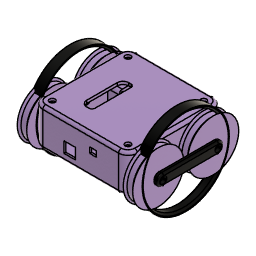
Bug (Autodesk Fusion 360 design; units mm, degrees)
Autodesk Fusion 360 part; units mm, degrees
sketch "Sketch1" plane through (0, 0, 0) normal (0, 0, 1) x (1, 0, 0)
  line L0 (-40, 50) -> (40, 50)
  line L1 (50, 40) -> (50, -40)
  line L2 (40, -50) -> (-40, -50)
  line L3 (-50, -40) -> (-50, 40)
  line L4 (-50, 0) -> (0, 0) construction
  line L5 (0, 50) -> (0, 0) construction
  arc A0 (-40, 50) -> (-50, 40) centre (-40, 40) ccw
  arc A1 (50, 40) -> (40, 50) centre (40, 40) ccw
  arc A2 (-50, -40) -> (-40, -50) centre (-40, -40) ccw
  arc A3 (40, -50) -> (50, -40) centre (40, -40) ccw
  arc A4 (47, 40) -> (40, 47) centre (40, 40) ccw
  line L6 (-40, 47) -> (40, 47)
  arc A5 (-40, 47) -> (-47, 40) centre (-40, 40) ccw
  line L7 (-47, -40) -> (-47, 40)
  arc A6 (-47, -40) -> (-40, -47) centre (-40, -40) ccw
  line L8 (40, -47) -> (-40, -47)
  arc A7 (40, -47) -> (47, -40) centre (40, -40) ccw
  line L9 (47, 40) -> (47, -40)
  circle A8 centre (23.9, -29.85) radius 1.4
  circle A9 centre (19.2, 22) radius 1.4
  circle A10 centre (-8.7, 22) radius 1.4
  circle A11 centre (-8.7, 22) radius 4
  circle A12 centre (19.2, 22) radius 4
  circle A13 centre (23.9, -29.85) radius 4
  line L10 (27.5, 47) -> (47, 27.5)
  line L11 (27.5, 47) -> (52.1887, 47) construction
  line L12 (-47, -27.5) -> (-27.5, -47)
  line L13 (-47, -27.5) -> (-27.798, -27.5) construction
  line L14 (27.5, -47) -> (47, -27.5)
  line L15 (27.5, -47) -> (53.0622, -47) construction
  line L16 (-27.5, 47) -> (-47, 27.5)
  line L17 (-27.5, 47) -> (-10.4675, 47) construction
  point P0 (-50, 50)
  point P1 (50, 50)
  point P2 (-50, -50)
  dimension "d1" = 100
  dimension "d2" = 100
  dimension "d3" = 10
  dimension "d4" = 10
  dimension "d5" = 10
  dimension "d6" = 10
  dimension "d7" = 3
  dimension "d8" = 2.8
  dimension "d9" = 2.8
  dimension "d10" = 2.8
  dimension "d11" = 20.15
  dimension "d12" = 72
  dimension "d13" = 26.1
  dimension "d14" = 30.8
  dimension "d15" = 27.9
  dimension "d16" = 8
  dimension "d17" = 8
  dimension "d18" = 8
  dimension "d19" = 45
  dimension "d20" = 45
  dimension "d21" = 45
  dimension "d22" = 135
  dimension "d23" = 22.5
  dimension "d24" = 22.5
  dimension "d25" = 22.5
  dimension "d26" = 22.5
  constraint horizontal L0
  constraint vertical L1
  constraint horizontal L2
  constraint vertical L3
  constraint coincident L4.end L5.end
  constraint vertical L5
  constraint horizontal L4
  constraint coincident L0 L5.start
  constraint coincident L3 L4.start
  constraint coincident P0 L0
  constraint coincident P0 L3
  constraint tangent L0 A0
  constraint tangent L3 A0
  constraint coincident P1 L0
  constraint coincident P1 L1
  constraint tangent L0 A1
  constraint tangent L1 A1
  constraint coincident P2 L2
  constraint coincident P2 L3
  constraint tangent L2 A2
  constraint tangent L3 A2
  constraint tangent L1 A3
  constraint tangent L2 A3
  constraint midpoint L0 L5.start
  constraint midpoint L3 L4.start
  constraint horizontal A9.centre A10.centre
  constraint concentric A10 A11
  constraint concentric A9 A12
  constraint concentric A8 A13
  constraint horizontal L11
  constraint coincident L6 L10.start
  constraint coincident L9 L10.end
  constraint horizontal L13
  constraint coincident L7 L12.start
  constraint coincident L8 L12.end
  constraint horizontal L15
  constraint coincident L8 L14.start
  constraint coincident L9 L14.end
  constraint horizontal L17
  constraint coincident L6 L16.start
  constraint coincident L7 L16.end
  measures "d1" distance of P0 P1
  measures "d2" distance of P0 P2
  measures "d3" radius of A0
  measures "d4" radius of A1
  measures "d5" radius of A2
  measures "d6" radius of A3
  measures "d8" diameter of A8
  measures "d9" diameter of A9
  measures "d10" diameter of A10
  measures "d11" distance of L2 A8.centre
  measures "d12" distance of L2 A9.centre
  measures "d13" distance of L1 A8.centre
  measures "d14" distance of L1 A9.centre
  measures "d15" distance of A9.centre A10.centre
  measures "d16" diameter of A11
  measures "d17" diameter of A12
  measures "d18" diameter of A13
  measures "d19" angle of L10 L11
  measures "d20" angle of L12 L13
  measures "d21" angle of L14 L15
  measures "d22" angle of L16 L17
  measures "d23" distance of L3 L16.start
  measures "d24" distance of L1 L10.start
  measures "d25" distance of L1 L14.start
  measures "d26" distance of L3 L12.end
extrude "Extrude2" add sketch "Sketch1" along normal blind 40 contours L0 L1 L2 L3 A0 A1 A2 A3 makes body 1
extrude "Extrude3" add sketch "Sketch1" along normal blind 3 contours L6 L7 L8 L9 L10 L12 L14 L16 bodies 1
extrude "Extrude4" add sketch "Sketch1" along normal blind 37 contours A4 L6 L9 L10 | L8 A7 L9 L14 | L6 A5 L7 L16 | L7 A6 L8 L12 bodies 1
extrude "Extrude5" add sketch "Sketch1" along normal blind 6 contours A11 | A12 | A13 bodies 1
extrude "Extrude6" add sketch "Sketch1" along normal blind 0.4 contours A8 | A9 | A10 bodies 1
fillet "Fillet3" radius 1 9 edges at (20.1707, -31.2965, 6) (22.5947, -29.3437, 6) (17.8947, 22.5063, 6) (15.4707, 20.5535, 6) (-10.0053, 22.5063, 6) (-12.4293, 20.5535, 6) (-12.4293, 23.4465, 3) (15.4707, 23.4465, 3) (20.1707, -28.4035, 3) on bodies 1
sketch "Sketch2" plane through (0, -50, 0) normal (0, -1, 0) x (1, 0, 0)
  line L0 (-40, 0) -> (40, 0)
  line L1 (40, 0) -> (40, 40)
  line L2 (40, 40) -> (-40, 40)
  line L3 (-40, 40) -> (-40, 0)
  line L4 (-17.7, 19.5) -> (-5.5, 19.5)
  line L5 (-5.5, 19.5) -> (-5.5, 8)
  line L6 (-5.5, 8) -> (-17.7, 8)
  line L7 (-17.7, 8) -> (-17.7, 19.5)
  line L8 (9.5, 27.5) -> (16.5, 27.5)
  line L9 (16.5, 27.5) -> (16.5, 21.5)
  line L10 (16.5, 21.5) -> (9.5, 21.5)
  line L11 (9.5, 21.5) -> (9.5, 27.5)
  line L12 (50, 0) -> (50, 40)
  dimension "d39" = 7
  dimension "d40" = 6
  dimension "d41" = 12.2
  dimension "d42" = 11.5
  dimension "d43" = 21.5
  dimension "d44" = 8
  dimension "d45" = 33.5
  dimension "d46" = 22
  dimension "d467" = 5.5
  constraint horizontal L4
  constraint vertical L5
  constraint horizontal L6
  constraint vertical L7
  constraint horizontal L8
  constraint vertical L9
  constraint horizontal L10
  constraint vertical L11
  measures "d39" distance of L8.start L8.end
  measures "d40" distance of L8.end L9.end
  measures "d41" distance of L4.start L4.end
  measures "d42" distance of L4.start L6.end
  measures "d43" distance of L0 L10
  measures "d44" distance of L0 L6
  measures "d45" distance of L9 L12
  measures "d46" distance of L5 L9
  measures "d467" distance of origin L5
extrude "Extrude7" cut sketch "Sketch2" against normal blind 10 contours L4 L5 L6 L7 | L8 L9 L10 L11 bodies 1
ref_plane "WorkPlane1" through (-37.25, -37.25, 29) normal (0, 0, 1) x (1, 0, 0)
sketch "Sketch5" plane through (-38.5, -38.5, 29) normal (0, 0, 1) x (1, 0, 0)
  line L0 (11, -8.5) -> (-8.5, 11)
  line L1 (78.5, -8.5) -> (-1.5, -8.5)
  arc A0 (-8.5, -1.5) -> (-1.5, -8.5) centre (-1.5, -1.5) ccw
  arc A1 (78.5, -8.5) -> (85.5, -1.5) centre (78.5, -1.5) ccw
  line L2 (85.5, 11) -> (66, -8.5)
  line L3 (85.5, 78.5) -> (85.5, -1.5)
  line L4 (-8.5, -1.5) -> (-8.5, 78.5)
extrude "Extrude8" cut sketch "Sketch5" against normal blind 26 bodies 1
ref_plane "WorkPlane2" through (0, -40.2, 21.5) normal (0, 1, 0) x (-1, 0, 0)
fillet "Fillet1" radius 3 6 edges at (47, -33.75, 29) (44.9497, -44.9497, 29) (33.75, -47, 29) (-33.75, -47, 29) (-44.9497, -44.9497, 29) (-47, -33.75, 29) on bodies 1
sketch "Sketch6" plane through (0, -40.2, 21.5) normal (0, 1, 0) x (1, 0, 0)
  line L0 (47, 18.5) -> (40, 18.5)
  line L1 (-40, 18.5) -> (-47, 18.5)
  line L2 (47, 18.5) -> (47, 4)
  line L3 (47, 4) -> (38.25, 4)
  line L4 (38.25, 4) -> (38.25, 10.5)
  line L5 (38.25, 10.5) -> (35.25, 10.5)
  line L6 (35.25, 10.5) -> (35.25, 4)
  line L7 (35.25, 4) -> (32.25, 4)
  line L8 (32.25, 4) -> (32.25, 18.5)
  line L9 (32.25, 18.5) -> (47, 18.5)
  dimension "d53" = 14.5
  dimension "d54" = 8.75
  dimension "d55" = 3
  dimension "d56" = 3
  dimension "d57" = 6.5
  constraint coincident L0.start L2.start
  constraint perpendicular L0 L2
  constraint perpendicular L2 L3
  constraint perpendicular L3 L4
  constraint perpendicular L2 L5
  constraint perpendicular L5 L6
  constraint perpendicular L2 L7
  constraint perpendicular L0 L8
  constraint perpendicular L2 L9
  constraint collinear L3 L7
  measures "d53" distance of L0.start L2.end
  measures "d54" distance of L2.end L3.end
  measures "d55" distance of L4.end L5.end
  measures "d56" distance of L6.end L7.end
  measures "d57" distance of L5.end L6.end
extrude "Extrude9" add sketch "Sketch6" against normal blind 6.8 bodies 1
fillet "Fillet2" radius 3 2 edges at (33.75, -40.2, 17.5) (42.6236, -40.2, 17.5) on bodies 1
sketch "Sketch7" plane through (47, 0, 0) normal (-1, 0, 0) x (0, -1, 0)
  line L0 (40, 26) -> (27.5, 26)
  line L1 (27.5, 26) -> (27.5, 37)
  line L2 (27.5, 37) -> (40, 37)
  line L3 (40, 37) -> (40, 40)
  line L4 (40, 40) -> (-40, 40)
  line L5 (-40, 40) -> (-40, 37)
  line L6 (-40, 37) -> (-27.5, 37)
  line L7 (-27.5, 37) -> (-27.5, 3)
  line L8 (-27.5, 3) -> (40, 3)
  line L9 (40, 3) -> (40, 26)
  circle A0 centre (29, 15) radius 6
  circle A1 centre (18, 15) radius 2.1
  line L10 (-5, 18) -> (-1, 18)
  line L11 (-1, 18) -> (-1, 12)
  line L12 (-1, 12) -> (-5, 12)
  line L13 (-5, 12) -> (-5, 18)
  line L14 (-25.5, 15) -> (-25.5, 3)
  line L15 (-32.5, 15) -> (-32.5, 3)
  line L16 (-32.5, 3) -> (-25.5, 3)
  arc A2 (-25.5, 15) -> (-32.5, 15) centre (-29, 15) ccw
  circle A3 centre (-29, 15) radius 1.4
  line L17 (50, 0) -> (50, 40)
  line L18 (-29, 18.5) -> (-40, 18.5)
  line L19 (-40, 18.5) -> (-40, 3)
  line L20 (-40, 3) -> (-32.5, 3)
  dimension "d66" = 12
  dimension "d67" = 4.2
  dimension "d68" = 4
  dimension "d69" = 6
  dimension "d70" = 7
  dimension "d71" = 2.8
  dimension "d72" = 12
  dimension "d73" = 9
  dimension "d74" = 12
  dimension "d75" = 11
  dimension "d76" = 21
  dimension "d77" = 19
  dimension "d78" = 47
  constraint horizontal L10
  constraint vertical L11
  constraint horizontal L12
  constraint vertical L13
  constraint coincident L8 L14.end
  constraint tangent L14 A2
  constraint perpendicular L8 L14
  constraint tangent L15 A2
  constraint perpendicular L8 L15
  constraint perpendicular L14 L16
  constraint concentric A2 A3
  constraint horizontal A0.centre A1.centre
  constraint midpoint A2 L18.start
  constraint tangent A2 L18
  constraint perpendicular L7 L18
  constraint perpendicular L16 L19
  constraint perpendicular L15 L20
  measures "d66" diameter of A0
  measures "d67" diameter of A1
  measures "d68" distance of L10.start L10.end
  measures "d69" distance of L10.start L12.end
  measures "d70" diameter of A2
  measures "d71" diameter of A3
  measures "d72" distance of L14.start L14.end
  measures "d73" distance of L8 L12
  measures "d74" distance of L8 A1.centre
  measures "d75" distance of A0.centre A1.centre
  measures "d76" distance of A0.centre L17
  measures "d77" distance of A1.centre L11
  measures "d78" distance of A1.centre A2.centre
extrude "Extrude10" cut sketch "Sketch7" along normal blind 3 and the other way blind 3 contours A0 | A3 bodies 1
extrude "Extrude11" cut sketch "Sketch7" against normal blind 2 contours A1 | L10 L11 L12 L13 bodies 1
extrude "Extrude12" add sketch "Sketch7" along normal blind 12 contours L7 L8 L14 L16 A2 | L7 L15 L16 A2 | L15 A2 L18 L19 L20 bodies 1
mirror "Mirror1" about plane through (0, 0, 0) normal (1, 0, 0) of "Extrude9", "Fillet2", "Extrude10", "Extrude11", "Extrude12"
fillet "Fillet5" radius 1 16 edges at (47, 5, 15) (47, 3, 18) (47, 1, 15) (47, 3, 12) (47, -16.0421, 15.7594) (50, -23.406, 12.8303) (47, -23.406, 17.1697) (-50, -23.406, 17.1697) (-47, -23.406, 12.8303) (-50, 30.3053, 15.5063) (-47, 3, 18) (-47, 5, 15) (-47, 3, 12) (-47, 1, 15) (-47, -16.0421, 14.2406) (50, 30.3053, 14.4937) on bodies 1
sketch "Sketch8" plane through (0, 0, 37) normal (0, 0, 1) x (-1, 0, 0)
  arc A0 (40, -47) -> (47, -40) centre (40, -40) ccw
  line L0 (47, -40) -> (47, -27.5)
  line L1 (47, -27.5) -> (27.5, -47)
  line L2 (27.5, -47) -> (40, -47)
  circle A1 centre (40, -40) radius 2.3
  circle A2 centre (-40, -40) radius 2.3
  circle A3 centre (-40, 40) radius 2.3
  circle A4 centre (40, 40) radius 2.3
  arc A5 (-47, -40) -> (-40, -47) centre (-40, -40) ccw
  arc A6 (-40, 47) -> (-47, 40) centre (-40, 40) ccw
  arc A7 (47, 40) -> (40, 47) centre (40, 40) ccw
  dimension "d94" = 4.6
  dimension "d95" = 4.6
  dimension "d96" = 4.6
  dimension "d97" = 4.6
  constraint concentric A0 A1
  constraint concentric A2 A5
  constraint concentric A3 A6
  constraint concentric A4 A7
  measures "d94" diameter of A1
  measures "d95" diameter of A2
  measures "d96" diameter of A3
  measures "d97" diameter of A4
extrude "Extrude13" cut sketch "Sketch8" against normal blind 5 contours A1 | A2 | A3 | A4 bodies 1
chamfer "Chamfer1" distance 0.75 distance2 1 4 edges at (-37.8556, 39.1683, 37) (42.1444, 39.1683, 37) (42.1444, -40.8317, 37) (-37.8556, -40.8317, 37) measured on face at (-35.2713, 45.1881, 37) measured on face at (35.2713, 45.1881, 37) measured on face at (35.2713, -45.1881, 37) measured on face at (-35.2713, -45.1881, 37) on bodies 1
sketch "Sketch9" plane through (0, 47, 0) normal (0, -1, 0) x (1, 0, 0)
  line L0 (-27.5, 37) -> (-27.5, 3)
  line L1 (-27.5, 3) -> (27.5, 3)
  line L2 (27.5, 3) -> (27.5, 37)
  line L3 (27.5, 37) -> (40, 37)
  line L4 (40, 37) -> (40, 40)
  line L5 (40, 40) -> (-40, 40)
  line L6 (-40, 40) -> (-40, 37)
  line L7 (-40, 37) -> (-27.5, 37)
  circle A0 centre (-13.2, 19.5) radius 8.2
  circle A1 centre (13.2, 19.5) radius 8.2
  line L8 (13.2, 19.5) -> (-13.2, 19.5) construction
  line L9 (0, 19.5) -> (0, 0) construction
  line L10 (-3.125, 14.375) -> (3.125, 14.375)
  line L11 (3.125, 10.625) -> (-3.125, 10.625)
  arc A2 (3.125, 10.625) -> (3.125, 14.375) centre (3.125, 12.5) ccw
  arc A3 (-3.125, 14.375) -> (-3.125, 10.625) centre (-3.125, 12.5) ccw
  dimension "d102" = 16.4
  dimension "d103" = 16.4
  dimension "d105" = 26.4
  dimension "d106" = 19.5
  dimension "d107" = 3.75
  dimension "d108" = 3.75
  dimension "d109" = 6.25
  dimension "d110" = 3.125
  dimension "d111" = 7
  constraint coincident A1.centre L8.start
  constraint coincident A0.centre L8.end
  constraint perpendicular L2 L8
  constraint midpoint L8 L9.start
  constraint coincident L9.end origin
  constraint vertical L9
  constraint tangent L10 A2
  constraint tangent L11 A3
  constraint perpendicular L9 L11
  constraint tangent L10 A3
  constraint tangent L11 A2
  measures "d102" diameter of A0
  measures "d103" diameter of A1
  measures "d105" distance of A1.centre A0.centre
  measures "d106" distance of L9.start L9.end
  measures "d107" diameter of A3
  measures "d108" diameter of A2
  measures "d109" distance of A3.centre A2.centre
  measures "d110" distance of L9 A2.centre
  measures "d111" vertical distance of A0.centre A3.centre
extrude "Extrude14" cut sketch "Sketch9" against normal blind 2 contours L10 L11 A2 A3 bodies 1
extrude "Extrude15" cut sketch "Sketch9" against normal blind 4 contours A0 | A1 bodies 1
fillet "Fillet6" radius 1 14 edges at (0, 47, 10.625) (-5, 47, 12.5) (0, 47, 14.375) (5, 47, 12.5) (5.5549, 47, 22.4652) (-20.8451, 47, 22.4652) (13, -47, 27.5) (9.5, -47, 24.5) (13, -47, 21.5) (16.5, -47, 24.5) (-5.5, -47, 13.75) (-11.6, -47, 19.5) (-17.7, -47, 13.75) (-11.6, -47, 8) on bodies 1
fillet "Fillet7" radius 3 16 edges at (0, -50, 40) (47.0711, -47.0711, 40) (50, 0, 40) (47.0711, 47.0711, 40) (0, 50, 40) (-47.0711, 47.0711, 40) (-50, 0, 40) (-47.0711, -47.0711, 40) (50, 0, 0) (47.0711, 47.0711, 0) (0, 50, 0) (-47.0711, 47.0711, 0) (-50, 0, 0) (-47.0711, -47.0711, 0) (0, -50, 0) (47.0711, -47.0711, 0) on bodies 1
sketch "Sketch10" plane through (0, 0, 37) normal (0, 0, 1) x (-1, 0, 0)
  arc A0 (47, 40) -> (40, 47) centre (40, 40) ccw
  line L0 (40, 47) -> (27.5, 47)
  line L1 (47, 27.5) -> (47, 40)
  circle A1 centre (40, 40) radius 3.05
  arc A2 (40, -47) -> (47, -40) centre (40, -40) ccw
  line L2 (40, -47) -> (-40, -47)
  line L3 (47, 40) -> (47, -40)
  arc A3 (47, 40) -> (40, 47) centre (40, 40) ccw
  line L4 (-40, 47) -> (40, 47)
  arc A4 (-40, 47) -> (-47, 40) centre (-40, 40) ccw
  line L5 (-47, -40) -> (-47, 40)
  arc A5 (-47, -40) -> (-40, -47) centre (-40, -40) ccw
  circle A6 centre (40, -40) radius 1.6
  circle A7 centre (-40, -40) radius 1.6
  circle A8 centre (-40, 40) radius 1.6
  circle A9 centre (40, 40) radius 1.6
  circle A10 centre (40, 40) radius 3
  circle A11 centre (-40, 40) radius 3
  circle A12 centre (-40, -40) radius 3
  circle A13 centre (40, -40) radius 3
  line L6 (13.5, 27.5) -> (16.2, 27.5)
  line L7 (22.2, 21.5) -> (22.2, -10.9)
  line L8 (16.2, -16.9) -> (13.5, -16.9)
  line L9 (10.5, -13.9) -> (10.5, 24.5)
  arc A14 (22.2, 21.5) -> (16.2, 27.5) centre (16.2, 21.5) ccw
  arc A15 (16.2, -16.9) -> (22.2, -10.9) centre (16.2, -10.9) ccw
  arc A16 (13.5, 27.5) -> (10.5, 24.5) centre (13.5, 24.5) ccw
  arc A17 (10.5, -13.9) -> (13.5, -16.9) centre (13.5, -13.9) ccw
  line L10 (10.5, -10.9) -> (1.5, -10.9)
  line L11 (1.5, -10.9) -> (1.5, -1.9)
  line L12 (1.5, -1.9) -> (10.5, -1.9)
  line L13 (10.5, -1.9) -> (10.5, -10.9)
  line L14 (10.5, 4.1) -> (1.5, 4.1)
  line L15 (1.5, 4.1) -> (1.5, 10.1)
  line L16 (1.5, 10.1) -> (10.5, 10.1)
  line L17 (10.5, 10.1) -> (10.5, 4.1)
  line L18 (10.5, 16.1) -> (1.5, 16.1)
  line L19 (1.5, 16.1) -> (1.5, 22.1)
  line L20 (1.5, 22.1) -> (10.5, 22.1)
  line L21 (10.5, 22.1) -> (10.5, 16.1)
  dimension "d120" = 3.2
  dimension "d121" = 3.2
  dimension "d122" = 3.2
  dimension "d123" = 3.2
  dimension "d124" = 6
  dimension "d125" = 6
  dimension "d126" = 6
  dimension "d127" = 6
  dimension "d208" = 11.7
  dimension "d209" = 44.4
  dimension "d210" = 19.5
  dimension "d211" = 24.8
  dimension "d212" = 6
  dimension "d213" = 6
  dimension "d214" = 3
  dimension "d215" = 3
  dimension "d316" = 9
  dimension "d317" = 6
  dimension "d318" = 9
  dimension "d410" = 6
  dimension "d411" = 6
  dimension "d412" = 6
  dimension "d413" = 6
  constraint concentric A2 A6
  constraint concentric A5 A7
  constraint concentric A4 A8
  constraint concentric A3 A9
  constraint concentric A3 A10
  constraint concentric A4 A11
  constraint concentric A5 A12
  constraint concentric A2 A13
  constraint horizontal L6
  constraint vertical L7
  constraint horizontal L8
  constraint vertical L9
  constraint tangent L6 A14
  constraint tangent L7 A14
  constraint tangent L7 A15
  constraint tangent L8 A15
  constraint tangent L6 A16
  constraint tangent L9 A16
  constraint tangent L8 A17
  constraint tangent L9 A17
  constraint horizontal L10
  constraint vertical L11
  constraint horizontal L12
  constraint vertical L13
  constraint coincident L9 L10.start
  constraint horizontal L14
  constraint vertical L15
  constraint horizontal L16
  constraint vertical L17
  constraint coincident L9 L14.start
  constraint horizontal L18
  constraint vertical L19
  constraint horizontal L20
  constraint vertical L21
  constraint coincident L9 L18.start
  constraint collinear L11 L15
  constraint collinear L15 L19
  measures "d120" diameter of A6
  measures "d121" diameter of A7
  measures "d122" diameter of A8
  measures "d123" diameter of A9
  measures "d124" diameter of A10
  measures "d125" diameter of A11
  measures "d126" diameter of A12
  measures "d127" diameter of A13
  measures "d208" distance of L7 L9
  measures "d209" distance of L6 L8
  measures "d210" distance of L4 L6
  measures "d211" distance of L3 L7
  measures "d212" radius of A14
  measures "d213" radius of A15
  measures "d214" radius of A16
  measures "d215" radius of A17
  measures "d316" distance of L10.end L11.end
  measures "d317" distance of L8 L10
  measures "d318" distance of L11.end L12.end
  measures "d410" distance of L14.end L15.end
  measures "d411" distance of L18.end L19.end
  measures "d412" distance of L12 L14
  measures "d413" distance of L16 L18
extrude "Extrude16" add sketch "Sketch10" along normal blind 3 separate body contours A0 L0 L1 A2 L2 L3 A3 L4 A4 L5 A5 | A1 | L9 L18 L19 L20 L21 | L9 L14 L15 L16 L17 | L9 L10 L11 L12 L13 makes body 2
extrude "Extrude17" add sketch "Sketch10" along normal blind 0.6 contours A10 | A11 | A12 | A13 bodies 2
chamfer "Chamfer2" distance 1 angle 45 8 edges at (0, 47, 37) (44.9497, 44.9497, 37) (47, 0, 37) (44.9497, -44.9497, 37) (0, -47, 37) (-44.9497, -44.9497, 37) (-47, 0, 37) (-44.9497, 44.9497, 37) on bodies 2
ref_plane "WorkPlane3" through (0, 0, 15) normal (0, 0, -1) x (-1, 0, 0)
sketch "Sketch11" plane through (0, 0, 15) normal (0, 0, -1) x (-1, 0, 0)
  line L0 (-51, 30.6) -> (-61, 30.6)
  line L1 (-61, 30.6) -> (-61, 56)
  line L2 (-51, 30.6) -> (-51, 56)
  line L3 (-51, 56) -> (-53, 54)
  line L4 (-53, 54) -> (-59, 54)
  line L5 (-59, 54) -> (-61, 56)
  line L6 (-50, 31.4) -> (-50, 26.6) construction
  line L7 (-50, -22) -> (-50, -36) construction
  line L8 (-61, -27.6) -> (-61, -2)
  line L9 (-61, -2) -> (-59, -4)
  line L10 (-59, -4) -> (-53, -4)
  line L11 (-53, -4) -> (-51, -2)
  line L12 (-51, -2) -> (-51, -24)
  line L13 (-51, -24) -> (-48, -24)
  line L14 (-48, -24) -> (-48, -27.6)
  line L15 (-50, -29) -> (-64.9565, -29) construction
  line L16 (-61, -27.6) -> (-48, -27.6)
  line L17 (-50, 29) -> (-62.9565, 29) construction
  line L18 (-50, 40) -> (-50, -40) construction
  line L19 (-50, -40) -> (-50, 40) construction
  line L20 (-50, 0) -> (-80, 0) construction
  line L21 (-61, -46) -> (-51, -46)
  line L22 (-51, -46) -> (-51, -45)
  line L23 (-51, -45) -> (-53, -43)
  line L24 (-53, -43) -> (-59, -43)
  line L25 (-59, -43) -> (-61, -45)
  line L26 (-61, -45) -> (-61, -46)
  dimension "d133" = 10
  dimension "d136" = 2
  dimension "d137" = 2
  dimension "d138" = 2
  dimension "d142" = 2
  dimension "d143" = 2
  dimension "d144" = 2
  dimension "d145" = 3
  dimension "d146" = 27
  dimension "d147" = 1.4
  dimension "d148" = 5
  dimension "d149" = 10
  dimension "d150" = 27
  dimension "d151" = 1.6
  dimension "d152" = 1
  dimension "d176" = 10
  dimension "d177" = 1
  dimension "d178" = 3
  dimension "d179" = 2
  dimension "d180" = 46
  constraint perpendicular L0 L1
  constraint perpendicular L0 L2
  constraint perpendicular L2 L4
  constraint vertical L2
  constraint perpendicular L8 L10
  constraint vertical L12
  constraint horizontal L8.end L11.end
  constraint collinear L1 L8
  constraint perpendicular L7 L13
  constraint perpendicular L13 L14
  constraint midpoint L7 L15.start
  constraint perpendicular L7 L15
  constraint midpoint L6 L17.start
  constraint perpendicular L6 L17
  constraint horizontal L1.end L2.end
  constraint midpoint L18 L20.start
  constraint perpendicular L18 L20
  constraint horizontal L21
  constraint vertical L22
  constraint perpendicular L22 L24
  constraint vertical L26
  constraint horizontal L22.end L25.end
  constraint equal L23 L25
  constraint collinear L8 L26
  measures "d133" distance of L0.start L0.end
  measures "d136" horizontal distance of L2.end L3.end
  measures "d137" vertical distance of L2.end L3.end
  measures "d138" horizontal distance of L1.end L4.end
  measures "d142" horizontal distance of L10.end L11.end
  measures "d143" vertical distance of L8.end L9.end
  measures "d144" horizontal distance of L8.end L9.end
  measures "d145" distance of L12.end L13.end
  measures "d146" distance of L8.end L15
  measures "d147" distance of L15 L16
  measures "d148" distance of L13 L15
  measures "d149" distance of L8 L12
  measures "d150" distance of L1.end L17
  measures "d151" distance of L0 L17
  measures "d152" distance of L2 L18
  measures "d176" distance of L21.start L21.end
  measures "d177" distance of L21.end L22.end
  measures "d178" distance of L21 L24
  measures "d179" horizontal distance of L24.end L25.end
  measures "d180" distance of L20 L21
revolve "Revolve1" add sketch "Sketch11" angle 360 about axis through (50, 29, 15) along (1, 0, 0) separate body contours L0 L1 L2 L3 L4 L5 makes body 3
revolve "Revolve2" add sketch "Sketch11" angle 360 about axis through (50, -29, 15) along (1, 0, 0) separate body contours L8 L9 L10 L11 L12 L13 L14 L16 makes body 4
revolve "Revolve3" add sketch "Sketch11" angle 360 about axis through (50, 0, 15) along (1, 0, 0) separate body contours L21 L22 L23 L24 L25 L26 makes body 5
sketch "Sketch12" plane through (48, 0, 0) normal (-1, 0, 0) x (0, -1, 0)
  circle A0 centre (29, 15) radius 5
  circle A1 centre (29, 15) radius 1.4
  circle A2 centre (29, 15) radius 2.8
  line L0 (27.0404, 17) -> (30.9596, 17)
  line L1 (30.9596, 13) -> (27.0404, 13)
  dimension "d155" = 5.6
  dimension "d156" = 4
  constraint concentric A0 A2
  constraint coincident A2 L0.start
  constraint coincident A2 L0.end
  constraint horizontal L0
  constraint coincident A2 L1.start
  constraint coincident A2 L1.end
  constraint parallel L0 L1
  constraint equal L0 L1
  measures "d155" diameter of A2
  measures "d156" distance of L0 L1
extrude "Extrude18" cut sketch "Sketch12" against normal blind 8 contours A2 L0 L1 bodies 4
fillet "Fillet8" radius 1 5 edges at (48, -29, 17) (48, -29, 13) (48, -26.2, 15) (48, -31.8, 15) (51, -30.8081, 10.3384) on bodies 4
ref_plane "WorkPlane4" through (61.5, -29, 15) normal (1, 0, 0) x (0, 0, -1)
sketch "Sketch13" plane through (61.5, -29, 15) normal (1, 0, 0) x (0, 1, 0)
  circle A0 centre (0, 0) radius 1.6
  circle A1 centre (58, 0) radius 1.6 construction
  circle A2 centre (58, 0) radius 1.6
  circle A3 centre (0, 0) radius 3.5
  circle A4 centre (58, 0) radius 3.5
  circle A5 centre (58, 0) radius 6
  circle A6 centre (0, 0) radius 6
  line L0 (0, 6) -> (58, 6)
  line L1 (0, -6) -> (58, -6)
  dimension "d162" = 3.2
  dimension "d163" = 3.2
  dimension "d164" = 7
  dimension "d165" = 7
  dimension "d166" = 12
  dimension "d167" = 12
  constraint coincident A0.centre A3.centre
  constraint concentric A1 A2
  constraint concentric A2 A4
  constraint concentric A4 A5
  constraint coincident A6 L0.start
  constraint coincident A5 L0.end
  constraint tangent A5 L0
  constraint coincident A6 L1.start
  constraint coincident A5 L1.end
  constraint tangent A5 L1
  constraint tangent A6 L0
  constraint tangent A6 L1
  measures "d162" diameter of A0
  measures "d163" diameter of A2
  measures "d164" diameter of A3
  measures "d165" diameter of A4
  measures "d166" diameter of A5
  measures "d167" diameter of A6
extrude "Extrude19" add sketch "Sketch13" along normal blind 5 separate body contours A5 | A5 A6 L0 L1 | A6 makes body 6
extrude "Extrude20" add sketch "Sketch13" along normal blind 1 contours A3 | A4 bodies 6
fillet "Fillet9" radius 2 4 edges at (66.5, 0, 9) (66.5, 35, 15) (66.5, 0, 21) (66.5, -35, 15) on bodies 6
fillet "Fillet9" radius 1 4 edges at (61.5, 0, 21) (61.5, -35, 15) (61.5, 0, 9) (61.5, 35, 15) on bodies 6
mirror "Mirror2" about plane through (0, 0, 0) normal (1, 0, 0) of bodies 4 6 3 5 makes body 7 at (-61, 47.4269, 13.5791) makes body 8 at (-61, -10.6339, 13.6586) makes body 9 at (-61.5, -9.1861, 18.5647) makes body 10 at (-57.6667, -45.9428, 17.2929)
equation "d411 = d410"
named bodies: "Body", "Lid", "Idle Wheel (R)", "Drive Wheel (R)", "Wheel Brace (R)", "Idle Wheel (L)", "Drive Wheel (L)", "Wheel Brace (L)", "Tread (R)", "Tread (L)"
